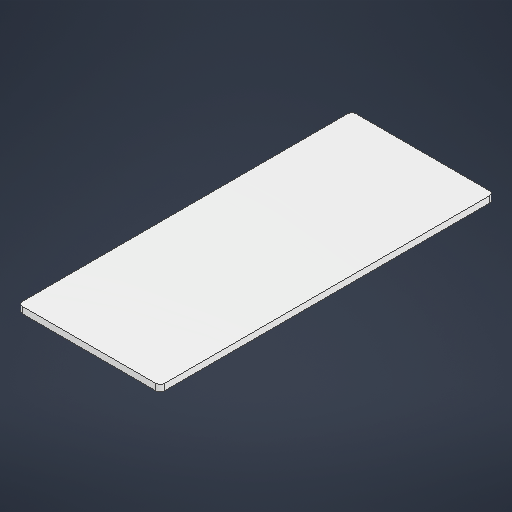
# Autodesk Inventor part: module-lid_switch
Saved by Autodesk Inventor 2025.2 (Build 292293000, 293)
## iProperties
Created: 2025-09-07
Part Number: module-lid_switch
Material: PC/ABS Plastic
Document SubType Name: Modeling
Designer: sam
Density: 1.1 g/cm^3
Appearance: Smooth - White
Author: sam
Autodesk Inventor part; units mm, degrees
ref_plane "YZ Plane" through (0, 0, 0) normal (1, 0, 0) x (0, 1, 0)
ref_plane "XZ Plane" through (0, 0, 0) normal (0, 1, 0) x (-1, 0, 0)
ref_plane "XY Plane" through (0, 0, 0) normal (0, 0, 1) x (1, 0, 0)
sketch "Sketch1" plane through (0, 0, 0) normal (0, 1, 0) x (-1, 0, 0)
  line L0 (-33.2, -78) -> (33.2, -78)
  line L1 (33.2, -78) -> (33.2, 78)
  line L2 (33.2, 78) -> (-33.2, 78)
  line L3 (-33.2, 78) -> (-33.2, -78)
  line L4 (-33.2, -78) -> (33.2, 78) construction
  line L5 (33.2, -78) -> (-33.2, 78) construction
  point P0 (0, 0)
  dimension "d0" = 66.4
  dimension "d1" = 156
  constraints: 12 end point, 2 midpoint, 2 parallel, 1 horizontal, 1 perpendicular
  measures "d0" distance of L2.end L1.end
  measures "d1" distance between parallel lines of L0 L2
extrude "Extrusion1" add sketch "Sketch1" along normal blind 3
sketch "Sketch2" plane through (0, 0, 0) normal (0, -1, 0) x (1, 0, 0)
  line L0 (30.2, 75) -> (-30.2, 75)
  line L1 (-30.2, 75) -> (-30.2, -75)
  line L2 (-30.2, -75) -> (30.2, -75)
  line L3 (30.2, -75) -> (30.2, 75)
  line L4 (30.2, 75) -> (-30.2, -75) construction
  line L5 (-30.2, 75) -> (30.2, -75) construction
  line L6 (-33.2, -78) -> (-33.2, 78) projected
  line L7 (33.2, -78) -> (-33.2, -78) projected
  point P0 (0, 0)
  dimension "d4" = 3
  dimension "d5" = 3
  constraints: 12 end point, 2 midpoint, 2 parallel, 1 horizontal, 1 perpendicular
  measures "d4" distance between parallel lines of L6 L1
  measures "d5" distance between parallel lines of L7 L2
extrude "Extrusion2" add sketch "Sketch2" along normal blind 3
fillet "Fillet1" radius 2 8 edges at (33.2, 1.5, 78) (30.2, -1.5, 75) (-30.2, -1.5, 75) (-33.2, 1.5, 78) (30.2, -1.5, -75) (33.2, 1.5, -78) (-33.2, 1.5, -78) (-30.2, -1.5, -75)
fillet "Fillet2" radius 0.5 8 edges at (-29.6142, -3, 74.4142) (-30.2, -3, 0) (-29.6142, -3, -74.4142) (0, -3, -75) (29.6142, -3, -74.4142) (30.2, -3, 0) (29.6142, -3, 74.4142) (0, -3, 75)
body "Solid1"
